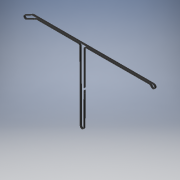
# Autodesk Inventor part: Part5
Saved by Autodesk Inventor 2018 (Build 220112000, 112)
## iProperties
Created: 2017-11-21
Part Number: Part5
Material: Rubber
Document SubType Name: Modeling
Designer: Gabriel Smolnycki
Density: 0.93 g/cm^3
Appearance: Rubber - Black
Author: Gabriel Smolnycki
Autodesk Inventor part; units mm, degrees
ref_plane "YZ Plane" through (0, 0, 0) normal (1, 0, 0) x (0, 1, 0)
ref_plane "XY Plane" through (0, 0, 0) normal (0, 0, 1) x (1, 0, 0)
sketch "Sketch1" plane through (0, 0, 0) normal (0, 0, 1) x (1, 0, 0)
  circle A0 centre (28, 14) radius 6.5 construction
  circle A1 centre (42.8324, 8) radius 6.5 construction
  circle A2 centre (203.5, 8) radius 6.5 construction
  circle A3 centre (232.5, 8) radius 6.5 construction
  circle A4 centre (492, 14) radius 7.5 construction
  circle A5 centre (477.1676, 8) radius 7.5 construction
  line L0 (226, -113.5) -> (226, -123.5) projected
  line L1 (226, -132.5) -> (226, -142.5) projected
  circle A6 centre (218, -258) radius 6.5 construction
  arc A7 (211.5, -258) -> (224.5, -258) centre (218, -258) ccw
  line L2 (211.5, -258) -> (210, 8)
  arc A8 (210, 8) -> (203.5, 14.5) centre (203.5, 8) ccw
  line L3 (203.5, 14.5) -> (42.8324, 14.5)
  line L4 (28, 20.5) -> (492, 21.5)
  line L5 (482.707, 13.0562) -> (486.4606, 8.9438)
  arc A9 (486.4606, 8.9438) -> (492, 21.5) centre (492, 14) ccw
  arc A10 (482.707, 13.0562) -> (477.1676, 15.5) centre (477.1676, 8) ccw
  line L6 (477.1676, 15.5) -> (232.5, 14.5)
  arc A11 (232.5, 14.5) -> (226, 8) centre (232.5, 8) ccw
  line L7 (226, 8) -> (226, -113.5)
  line L8 (224.5, -258) -> (226, -142.5)
  arc A12 (5.8911, 2.4402) -> (5.3018, 3.5426) centre (0, 0) ccw projected
  arc A13 (-2.8741, 5.692) -> (3.3144, -5.4474) centre (0, 0) ccw
  line L9 (-2.8741, 5.692) -> (25.0702, 19.8023)
  line L10 (3.3144, -5.4474) -> (30.5, 8)
  line L11 (39.3575, 13.4932) -> (31.4749, 8.5068)
  arc A14 (42.8324, 14.5) -> (39.3575, 13.4932) centre (42.8324, 8) ccw
  arc A15 (30.5, 8) -> (31.4749, 8.5068) centre (28, 14) ccw
  arc A16 (28, 20.5) -> (25.0702, 19.8023) centre (28, 14) ccw
  point P0 (0, 0)
  dimension "d2" = 6.3764
  dimension "d3" = 12.7529
  constraints: 34 point on circle, 20 end point, 9 centre point, 9 coincident, 6 tangent, 4 concentric, 1 collinear, 1 horizontal
  measures "d2" radius of A12
  measures "d3" diameter of A13
ref_plane "Work Plane1" through (226, -123.5, 0) normal (0, 1, 0) x (-1, 0, 0)
sketch "Sketch2" plane through (226, -123.5, 0) normal (0, 1, 0) x (-1, 0, 0)
  line L0 (0.65, -3) -> (-0.65, -3)
  line L1 (-0.65, -3) -> (-0.65, 3)
  line L2 (-0.65, 3) -> (0.65, 3)
  line L3 (0.65, 3) -> (0.65, -3)
  line L4 (0.65, -3) -> (-0.65, 3) construction
  line L5 (-0.65, -3) -> (0.65, 3) construction
  point P0 (226, 0)
  point P1 (0, 0)
  point P2 (0, 0)
  point P3 (0, 0)
  dimension "d0" = 1.3
  dimension "d1" = 6
  constraints: 12 end point, 3 midpoint, 2 parallel, 1 coincident, 1 horizontal, 1 perpendicular
  measures "d0" distance of L1.end L2.end
  measures "d1" distance of L0.end L1.end
sweep "Sweep1" add profiles "Sketch2" path "Sketch1" path curves L0 L7 A11 L6 A10 L5 A9 L4 A16 L9 A13 L10 A15 L11 A14 L3 A8 L2 A7 L8 L1
equation "\"d3\" = 2 * d2"
body "Solid1"
